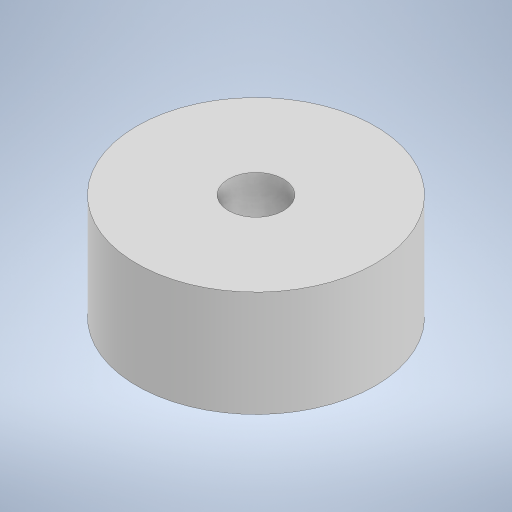
# Autodesk Inventor part: 4. ring
Saved by Autodesk Inventor 2024 (Build 280153000, 153)
## iProperties
Created: 2024-02-22
Part Number: 4. ring
Material: Generic
Document SubType Name: Modeling
Designer: evmgm
Density: 1 g/cm^3
Appearance: Default
Author: evmgm
Autodesk Inventor part; units mm, degrees
ref_plane "YZ Plane" through (0, 0, 0) normal (1, 0, 0) x (0, 1, 0)
ref_plane "XZ Plane" through (0, 0, 0) normal (0, 1, 0) x (-1, 0, 0)
ref_plane "XY Plane" through (0, 0, 0) normal (0, 0, 1) x (1, 0, 0)
sketch "Sketch1" plane through (0, 0, 0) normal (0, 1, 0) x (-1, 0, 0)
  circle A0 centre (0, 0) radius 22.5
  circle A1 centre (0, 0) radius 12.7
  circle A2 centre (0, 0) radius 5.2
  dimension "d1" = 45
  dimension "d14" = 25.4
  dimension "d15" = 10.4
  constraints: 3 centre point, 2 coincident
  measures "d1" diameter of A0
  measures "d14" diameter of A1
  measures "d15" diameter of A2
extrude "Extrusion1" add sketch "Sketch1" along normal blind 20 contours A0 | A1 | A2
extrude "Extrusion2" cut sketch "Sketch1" along normal blind 11.4 contours A1
extrude "Extrusion3" cut sketch "Sketch1" along normal blind 20 contours A2
chamfer "Chamfer2" distance 11.4 distance2 7.5 1 edges at (12.7, 11.4, 0) measured on face at (-12.5355, 7.6, -2.0372)
body "Solid1"
